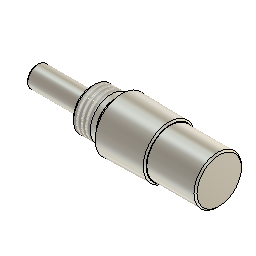
SKM-88 v1 (Autodesk Fusion 360 design; units mm, degrees)
Autodesk Fusion 360 part; units mm, degrees
sketch "Sketch1" plane through (0, 0, 0) normal (0, 0, 1) x (1, 0, 0)
  line L0 (0, 0) -> (30, 0)
  line L1 (9, 0) -> (9, 3.5)
  line L2 (9, 3.5) -> (14, 3.5)
  line L3 (14, 3.5) -> (14, 4.4)
  line L4 (14, 4.4) -> (22, 4.4) construction
  line L5 (22, 4.4) -> (22, 0) construction
  line L6 (22, 0) -> (22, 4.25) construction
  line L7 (22, 4.25) -> (14, 4.4)
  line L8 (22, 4.25) -> (22, 0)
  line L9 (0, 0) -> (0, 1.75) construction
  line L10 (0, 1.75) -> (9, 1.75) construction
  line L11 (8.5, 1.75) -> (8.5, 2.25)
  line L12 (8.5, 2.25) -> (9, 2.25)
  line L13 (8.5, 1.75) -> (0, 1.75)
  line L14 (0, 1.75) -> (0, 0)
  line L15 (9, 1.75) -> (30, 1.75)
  line L16 (30, 1.75) -> (30, 0)
  line L17 (30, 0) -> (30, 3.9)
  line L18 (30, 3.9) -> (22, 3.9)
  line L19 (14, 0) -> (14, 2.9)
  line L20 (14, 2.9) -> (14, 3.5)
  line L21 (14, 2.9) -> (12.75, 2.9)
  line L22 (12.75, 2.9) -> (12.75, 3.5)
  dimension "d1" = 30
  dimension "d2" = 9
  dimension "d3" = 3.5
  dimension "d4" = 5
  dimension "d5" = 4.4
  dimension "d6" = 8
  dimension "d7" = 4.25
  dimension "d8" = 1.75
  dimension "d9" = 2.25
  dimension "d10" = 0.5
  dimension "d11" = 3.9
  dimension "d12" = 90
  dimension "d15" = 2.9
  dimension "d16" = 1.25
  constraint coincident L0.start L9.start
  constraint horizontal L0
  constraint coincident L0 L1.start
  constraint perpendicular L0 L1
  constraint perpendicular L1 L2
  constraint perpendicular L0 L3
  constraint perpendicular L3 L4
  constraint coincident L0 L5.end
  constraint perpendicular L0 L5
  constraint coincident L5 L6.end
  constraint perpendicular L0 L9
  constraint midpoint L1 L10.end
  constraint coincident L10 L11.start
  constraint perpendicular L10 L11
  constraint coincident L1 L12.end
  constraint perpendicular L1 L12
  constraint perpendicular L1 L15
  constraint coincident L0 L16.end
  constraint perpendicular L0 L16
  constraint coincident L0.end L16.end
  constraint perpendicular L0 L17
  constraint coincident L8 L18.end
  constraint coincident L0 L19.start
  constraint perpendicular L0 L19
  constraint vertical L20
  constraint perpendicular L19 L21
  constraint coincident L2 L22.end
  constraint perpendicular L2 L22
  measures "d1" distance of L0.start L0.end
  measures "d2" distance of L0.start L1.start
  measures "d3" distance of L1.start L1.end
  measures "d4" distance of L1.end L2.end
  measures "d5" distance of L0 L3.end
  measures "d6" distance of L3.end L4.end
  measures "d7" distance of L5.end L6.end
  measures "d8" distance of L0.start L9.end
  measures "d9" distance of L0 L11.end
  measures "d10" distance of L1 L11.end
  measures "d11" distance of L0.end L17.end
  measures "d12" angle of L17 L18
  measures "d15" distance of L19.start L19.end
  measures "d16" distance of L19.end L21.end
revolve "Revolve1" add sketch "Sketch1" angle 360 about axis through (0, 0, 0) along (1, 0, 0) contours L0 L1 L15 L19 | L0 L8 L15 L19 | L1 L2 L15 L19 L21 L22 | L3 L7 L8 L15 L19 L20 makes body 1
revolve "Revolve2" add sketch "Sketch1" angle 360 about axis through (0, 0, 0) along (1, 0, 0) separate body contours L0 L1 L11 L12 L13 L14 | L0 L1 L15 L19 | L0 L8 L15 L19 | L0 L8 L15 L16 L17 | L8 L15 L17 L18 makes body 2
thread "Thread1" "ISO Metric profile 7.0 M7x0.75 6g" major diameter 6.908 minor diameter 6.0475 pitch 0.75 angle 60 resizes the face on face at (10.25, 3.4826, -0.3485) on bodies 1
copy_body "Body->Comp1" bodies 1 removing the originals makes body 3 in component "Body"
copy_body "Body->Comp2" bodies 2 removing the originals makes body 4 in component "Plunger"
chamfer "Chamfer1" distance 0.25 angle 45 1 edges at (30, -1.4103, 3.6361) on bodies 4 in component "Plunger"
chamfer "Chamfer1'" distance 0.25 angle 45 1 edges at (22, -1.5369, 3.9624) on bodies 3 in component "Body"
chamfer "Chamfer2" distance 0.25 angle 45 1 edges at (0, -0.6328, 1.6316) on bodies 4 in component "Plunger"
chamfer "Chamfer2'" distance 0.5 angle 45 1 edges at (9, -3.2203, -1.249) on bodies 3 in component "Body"
chamfer "Chamfer3" distance 0.5 angle 45 1 edges at (12.75, -3.2203, -1.249) on bodies 3 in component "Body"
component "Body" placed x (1, 0, 0) y (0, 1, 0) z (0, 0, 1) at (0, 0, 0)
component "Plunger" placed x (1, 0, 0) y (0, 1, 0) z (0, 0, 1) at (0, 0, 0)
equation "d3 = ( 7 / 2 ) * 1 mm"
equation "d5 = 8.8 mm / 2"
equation "d7 = ( 8.5 / 2 ) * 1 mm"
equation "d8 = 3.5 mm / 2"
equation "d9 = ( 4.5 / 2 ) * 1 mm"
equation "d11 = ( 7.8 / 2 ) * 1 mm"
equation "d15 = ( 5.8 / 2 ) * 1 mm"
named bodies: "Body", "Plunger"
